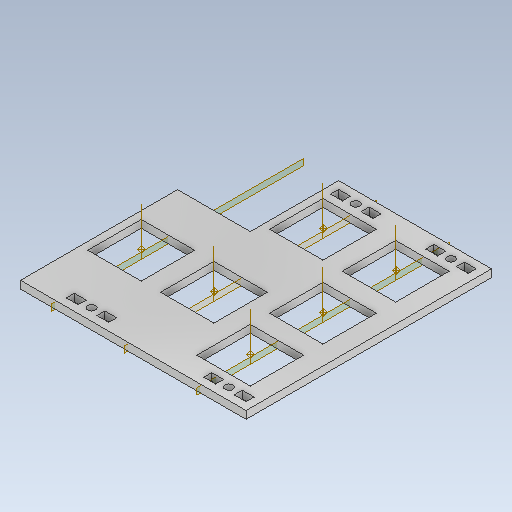
# Autodesk Inventor part: tc_base_plate
Saved by Autodesk Inventor 2020.1 (Build 241239000, 239)
## iProperties
Created: 2019-07-03
Part Number: tc_base_plate
Material: Acier inoxydable
Document SubType Name: Modeling
Designer: Thibault
Density: 8 g/cm^3
Appearance: Aluminium - Poli
Mass: 33.3223 g
Surface Area: 56.2435 cm^2
Volume: 4.16528 cm^3
tc_base_width: 59,100 mm
tc_base_back_width: 40,050 mm
tc_base_support_dist: 56,100 mm
Author: Thibault
Autodesk Inventor part; units mm, degrees
ref_plane "YZ Plane" through (0, 0, 0) normal (1, 0, 0) x (0, 1, 0)
ref_plane "XZ Plane" through (0, 0, 0) normal (0, 1, 0) x (-1, 0, 0)
ref_plane "XY Plane" through (0, 0, 0) normal (0, 0, 1) x (1, 0, 0)
sketch "screw_anchor" plane through (0, 0, 0) normal (0, 0, 1) x (1, 0, 0)
  point P0 (61.1245, 15.5217)
  dimension "d155" = 14
  dimension "d156" = 19.05
  dimension "d157" = 19.05
  dimension "d158" = 19.05
  dimension "d159" = 28.575
  dimension "d160" = 19.05
  dimension "d161" = 2
  dimension "d162" = 2
  dimension "d163" = 2
  dimension "d164" = 2
  dimension "d165" = 2
  dimension "d166" = 1
  dimension "d167" = 5
  dimension "d168" = 5
  dimension "d169" = 4
  dimension "tc_base_support_dist" = 56.1
sketch "anchor" plane through (0, 0, 0) normal (0, 0, 1) x (1, 0, 0)
  circle A0 centre (94.2814, 48.5827) radius 0.85
  line L0 (91.2814, 49.5827) -> (87.2814, 49.5827)
  line L1 (87.2814, 49.5827) -> (87.2814, 47.5827)
  line L2 (87.2814, 47.5827) -> (91.2814, 47.5827)
  line L3 (91.2814, 47.5827) -> (91.2814, 49.5827)
  line L4 (101.2814, 49.5827) -> (97.2814, 49.5827)
  line L5 (97.2814, 49.5827) -> (97.2814, 47.5827)
  line L6 (97.2814, 47.5827) -> (101.2814, 47.5827)
  line L7 (101.2814, 47.5827) -> (101.2814, 49.5827)
  line L8 (91.2814, 49.5827) -> (97.2814, 47.5827) construction
  line L9 (97.2814, 49.5827) -> (91.2814, 47.5827) construction
  line L10 (87.2814, 51.1827) -> (101.2814, 51.1827)
  point P0 (103.5798, 50.1132)
  point P1 (94.2814, 48.5827)
  dimension "tc_base_support_dist" = 56.1
  dimension "d226" = 1.7
  dimension "d230" = 4
  dimension "d231" = 2
  dimension "d237" = 4
  dimension "d245" = 1.6
  dimension "d247" = 6
  measures "d226" diameter of A0
  measures "d230" distance of L2.end L1.end
  measures "d231" distance of L1.end L0.end
  measures "d237" distance of L6.end L5.end
  measures "d245" distance between parallel lines of L0 L10
  measures "d247" distance between parallel lines of L5 L3
sketch "Anchor (screw side)" plane through (0, 0, 0) normal (0, 0, 1) x (1, 0, 0)
  circle A0 centre (93.7216, 50.3096) radius 1.05
  line L0 (91.2716, 51.3596) -> (88.1716, 51.3596)
  line L1 (88.1716, 51.3596) -> (88.1716, 49.2596)
  line L2 (88.1716, 49.2596) -> (91.2716, 49.2596)
  line L3 (91.2716, 49.2596) -> (91.2716, 51.3596)
  line L4 (99.2716, 51.3596) -> (96.1716, 51.3596)
  line L5 (96.1716, 51.3596) -> (96.1716, 49.2596)
  line L6 (96.1716, 49.2596) -> (99.2716, 49.2596)
  line L7 (99.2716, 49.2596) -> (99.2716, 51.3596)
  line L8 (91.2716, 51.3596) -> (96.1716, 49.2596) construction
  line L9 (96.1716, 51.3596) -> (91.2716, 49.2596) construction
  line L10 (86.1716, 53.3596) -> (101.2716, 53.3596) construction
  line L11 (101.2716, 53.3596) -> (101.2716, 47.2596) construction
  line L12 (101.2716, 47.2596) -> (86.1716, 47.2596) construction
  line L13 (86.1716, 47.2596) -> (86.1716, 53.3596) construction
  point P0 (103.5798, 50.1132)
  dimension "d27" = 2.1
  dimension "d28" = 3.1
  dimension "d29" = 2.1
  dimension "d32" = 4.9
  dimension "d34" = 2
  dimension "d35" = 2
  dimension "d36" = 2
  dimension "d37" = 2
  measures "d27" diameter of A0
  measures "d28" distance of L2.end L1.end
  measures "d29" distance of L1.end L0.end
  measures "d32" distance between parallel lines of L5 L3
  measures "d34" distance between parallel lines of L0 L10
  measures "d35" distance between parallel lines of L12 L2
  measures "d36" distance between parallel lines of L11 L7
  measures "d37" distance between parallel lines of L13 L1
sketch "Anchor (nut side)" plane through (0, 0, 0) normal (0, 0, 1) x (1, 0, 0)
  line L0 (10, 0) -> (8.55, 0)
  line L1 (8.55, 0) -> (8.55, -2)
  line L2 (8.55, -2) -> (9.35, -2)
  line L3 (9.35, -2) -> (9.35, -4)
  line L4 (5.65, -4) -> (5.65, -2)
  line L5 (5.65, -2) -> (6.45, -2)
  line L6 (6.45, -2) -> (6.45, 0)
  line L7 (6.45, 0) -> (5, 0)
  line L8 (2, 0) -> (2, 2)
  line L9 (2, 0) -> (3, 0) construction
  line L10 (2, 2) -> (5, 2)
  line L11 (5, 2) -> (5, 0)
  line L12 (10, 0) -> (10, 2)
  line L13 (10, 2) -> (13, 2)
  line L14 (13, 2) -> (13, 0)
  line L15 (0, 0) -> (2, 0)
  line L16 (13, 0) -> (15, 0)
  line L17 (5.65, -4) -> (6.45, -4)
  line L18 (9.35, -4) -> (8.55, -4)
  line L19 (6.45, -4) -> (6.45, -6.25)
  line L20 (8.55, -4) -> (8.55, -6.25)
  line L21 (6.7, -6.5) -> (7.5, -6.5)
  arc A0 (6.45, -6.25) -> (6.7, -6.5) centre (6.7, -6.25) ccw
  arc A1 (8.3, -6.5) -> (8.55, -6.25) centre (8.3, -6.25) ccw
  line L22 (7.5, -6.5) -> (8.3, -6.5)
  line L23 (7.5, -3.8983) -> (7.5, -9.959) construction
  point P0 (9.1321, -0.6227)
  point P1 (6.45, -6.5)
  point P2 (8.55, -6.5)
  dimension "d3" = 2
  dimension "d7" = 5
  dimension "d10" = 1.45
  dimension "d11" = 2
  dimension "d12" = 0.8
  dimension "d13" = 2
  dimension "d14" = 0.8
  dimension "d15" = 2.1
  dimension "d18" = 2
  dimension "d19" = 0.8
  dimension "d20" = 0.8
  dimension "d21" = 2.5
  dimension "d22" = 2.5
  dimension "d23" = 2.1
  dimension "d38" = 2
  dimension "d39" = 0.25
  dimension "d120" = 3
  measures "d3" distance of L15.start L8.start
  measures "d7" distance of L7.end L0.start
  measures "d10" distance of L0.start L0.end
  measures "d11" distance of L0.end L1.end
  measures "d12" distance of L1.end L2.end
  measures "d13" distance of L2.end L3.end
  measures "d14" distance of L4.end L5.end
  measures "d15" distance of L6.end L0.end
  measures "d18" distance of L14.end L16.end
  measures "d19" distance of L4.start L17.end
  measures "d20" distance of L3.end L18.end
  measures "d21" distance of L17.end point (6.45, -6.5)
  measures "d22" distance of L18.end point (8.55, -6.5)
  measures "d23" distance of L17.end L18.end
  measures "d38" distance between parallel lines of L15 L10
  measures "d39" radius of A0
  measures "d120" distance of L8.end L10.end
sketch "Screwless anchor (male)" plane through (0, 0, 0) normal (0, 0, 1) x (1, 0, 0)
  line L0 (2, 0) -> (2, 2)
  line L1 (2, 0) -> (3, 0) construction
  line L2 (2, 2) -> (5, 2)
  line L3 (5, 2) -> (5, 0)
  line L4 (10, 0) -> (10, 2)
  line L5 (10, 2) -> (13, 2)
  line L6 (13, 2) -> (13, 0)
  line L7 (0, 0) -> (2, 0)
  line L8 (13, 0) -> (15, 0)
  line L9 (5, 0) -> (10, 0)
  point P0 (9.1321, -0.6227)
  dimension "d81" = 2
  dimension "d83" = 5
  dimension "d92" = 2
  dimension "d100" = 2
  dimension "d119" = 3
  measures "d81" distance of L7.start L0.start
  measures "d83" distance of L3.end L4.start
  measures "d92" distance of L6.end L8.end
  measures "d100" distance between parallel lines of L7 L2
  measures "d119" distance of L0.end L2.end
sketch "Screwless anchor (female)" plane through (0, 0, 0) normal (0, 0, 1) x (1, 0, 0)
  line L0 (91.7814, 51.7592) -> (88.6814, 51.7592)
  line L1 (88.6814, 51.7592) -> (88.6814, 49.6592)
  line L2 (88.6814, 49.6592) -> (91.7814, 49.6592)
  line L3 (91.7814, 49.6592) -> (91.7814, 51.7592)
  line L4 (99.7814, 51.7592) -> (96.6814, 51.7592)
  line L5 (96.6814, 51.7592) -> (96.6814, 49.6592)
  line L6 (96.6814, 49.6592) -> (99.7814, 49.6592)
  line L7 (99.7814, 49.6592) -> (99.7814, 51.7592)
  line L8 (86.6814, 53.7592) -> (101.7814, 53.7592) construction
  line L9 (101.7814, 53.7592) -> (101.7814, 47.6592) construction
  line L10 (101.7814, 47.6592) -> (86.6814, 47.6592) construction
  line L11 (86.6814, 47.6592) -> (86.6814, 53.7592) construction
  point P0 (103.5798, 50.1132)
  dimension "d106" = 3.1
  dimension "d107" = 2.1
  dimension "d108_1" = 3.1
  dimension "d109_1" = 4.9
  dimension "d110_1" = 2
  dimension "d111_1" = 2
  dimension "d112" = 2
  dimension "d113" = 2
  measures "d106" distance of L2.end L1.end
  measures "d107" distance of L1.end L0.end
  measures "d108_1" distance of L6.end L5.end
  measures "d109_1" distance between parallel lines of L5 L3
  measures "d110_1" distance between parallel lines of L0 L8
  measures "d111_1" distance between parallel lines of L10 L2
  measures "d112" distance between parallel lines of L9 L7
  measures "d113" distance between parallel lines of L11 L1
sketch "Esquisse2" plane through (0, 0, 0) normal (0, 1, 0) x (-1, 0, 0)
  line L0 (17.4004, -3.6293) -> (3.4004, -3.6293)
  line L1 (3.4004, -3.6293) -> (3.4004, 10.3707)
  line L2 (3.4004, 10.3707) -> (17.4004, 10.3707)
  line L3 (17.4004, 10.3707) -> (17.4004, -3.6293)
  line L4 (17.4004, -41.7293) -> (3.4004, -41.7293)
  line L5 (3.4004, -41.7293) -> (3.4004, -27.7293)
  line L6 (3.4004, -27.7293) -> (17.4004, -27.7293)
  line L7 (17.4004, -27.7293) -> (17.4004, -41.7293)
  line L8 (17.4004, -22.6793) -> (3.4004, -22.6793)
  line L9 (3.4004, -22.6793) -> (3.4004, -8.6793)
  line L10 (3.4004, -8.6793) -> (17.4004, -8.6793)
  line L11 (17.4004, -8.6793) -> (17.4004, -22.6793)
  line L12 (36.4504, -41.7293) -> (22.4504, -41.7293)
  line L13 (22.4504, -41.7293) -> (22.4504, -27.7293)
  line L14 (22.4504, -27.7293) -> (36.4504, -27.7293)
  line L15 (36.4504, -27.7293) -> (36.4504, -41.7293)
  line L16 (36.4504, -13.1543) -> (22.4504, -13.1543)
  line L17 (22.4504, -13.1543) -> (22.4504, 0.8457)
  line L18 (22.4504, 0.8457) -> (36.4504, 0.8457)
  line L19 (36.4504, 0.8457) -> (36.4504, -13.1543)
  line L20 (55.5004, -13.1543) -> (41.5004, -13.1543)
  line L21 (41.5004, -13.1543) -> (41.5004, 0.8457)
  line L22 (41.5004, 0.8457) -> (55.5004, 0.8457)
  line L23 (55.5004, 0.8457) -> (55.5004, -13.1543)
  line L24 (57.5004, -24.6793) -> (38.4504, -24.6793)
  line L25 (38.4504, -24.6793) -> (38.4504, -47.8293)
  line L26 (38.4504, -47.8293) -> (-1.5996, -47.8293)
  line L27 (-1.5996, -47.8293) -> (-1.5996, 16.4707)
  line L28 (57.5004, -24.6793) -> (57.5004, 16.4707)
  line L29 (57.5004, 16.4707) -> (-1.5996, 16.4707)
  circle A0 centre (41.9504, 13.4207) radius 1.05
  line L30 (39.5004, 14.4707) -> (36.4004, 14.4707)
  line L31 (36.4004, 14.4707) -> (36.4004, 12.3707)
  line L32 (36.4004, 12.3707) -> (39.5004, 12.3707)
  line L33 (39.5004, 12.3707) -> (39.5004, 14.4707)
  line L34 (47.5004, 14.4707) -> (44.4004, 14.4707)
  line L35 (44.4004, 14.4707) -> (44.4004, 12.3707)
  line L36 (44.4004, 12.3707) -> (47.5004, 12.3707)
  line L37 (47.5004, 12.3707) -> (47.5004, 14.4707)
  line L38 (39.5004, 14.4707) -> (44.4004, 12.3707) construction
  line L39 (44.4004, 14.4707) -> (39.5004, 12.3707) construction
  line L40 (34.4004, 16.4707) -> (49.5004, 16.4707) construction
  line L41 (49.5004, 16.4707) -> (49.5004, 10.3707) construction
  line L42 (49.5004, 10.3707) -> (34.4004, 10.3707) construction
  line L43 (34.4004, 10.3707) -> (34.4004, 16.4707) construction
  circle A1 centre (5.9504, 13.4207) radius 1.05
  line L44 (3.5004, 14.4707) -> (0.4004, 14.4707)
  line L45 (0.4004, 14.4707) -> (0.4004, 12.3707)
  line L46 (0.4004, 12.3707) -> (3.5004, 12.3707)
  line L47 (3.5004, 12.3707) -> (3.5004, 14.4707)
  line L48 (11.5004, 14.4707) -> (8.4004, 14.4707)
  line L49 (8.4004, 14.4707) -> (8.4004, 12.3707)
  line L50 (8.4004, 12.3707) -> (11.5004, 12.3707)
  line L51 (11.5004, 12.3707) -> (11.5004, 14.4707)
  line L52 (3.5004, 14.4707) -> (8.4004, 12.3707) construction
  line L53 (8.4004, 14.4707) -> (3.5004, 12.3707) construction
  line L54 (-1.5996, 16.4707) -> (13.5004, 16.4707) construction
  line L55 (13.5004, 16.4707) -> (13.5004, 10.3707) construction
  line L56 (13.5004, 10.3707) -> (-1.5996, 10.3707) construction
  line L57 (-1.5996, 10.3707) -> (-1.5996, 16.4707) construction
  circle A2 centre (5.9504, -44.7793) radius 1.05
  line L58 (3.5004, -43.7293) -> (0.4004, -43.7293)
  line L59 (0.4004, -43.7293) -> (0.4004, -45.8293)
  line L60 (0.4004, -45.8293) -> (3.5004, -45.8293)
  line L61 (3.5004, -45.8293) -> (3.5004, -43.7293)
  line L62 (11.5004, -43.7293) -> (8.4004, -43.7293)
  line L63 (8.4004, -43.7293) -> (8.4004, -45.8293)
  line L64 (8.4004, -45.8293) -> (11.5004, -45.8293)
  line L65 (11.5004, -45.8293) -> (11.5004, -43.7293)
  line L66 (3.5004, -43.7293) -> (8.4004, -45.8293) construction
  line L67 (8.4004, -43.7293) -> (3.5004, -45.8293) construction
  line L68 (-1.5996, -41.7293) -> (13.5004, -41.7293) construction
  line L69 (13.5004, -41.7293) -> (13.5004, -47.8293) construction
  line L70 (13.5004, -47.8293) -> (-1.5996, -47.8293) construction
  line L71 (-1.5996, -47.8293) -> (-1.5996, -41.7293) construction
  circle A3 centre (30.9004, -44.7793) radius 1.05
  line L72 (28.4504, -43.7293) -> (25.3504, -43.7293)
  line L73 (25.3504, -43.7293) -> (25.3504, -45.8293)
  line L74 (25.3504, -45.8293) -> (28.4504, -45.8293)
  line L75 (28.4504, -45.8293) -> (28.4504, -43.7293)
  line L76 (36.4504, -43.7293) -> (33.3504, -43.7293)
  line L77 (33.3504, -43.7293) -> (33.3504, -45.8293)
  line L78 (33.3504, -45.8293) -> (36.4504, -45.8293)
  line L79 (36.4504, -45.8293) -> (36.4504, -43.7293)
  line L80 (28.4504, -43.7293) -> (33.3504, -45.8293) construction
  line L81 (33.3504, -43.7293) -> (28.4504, -45.8293) construction
  line L82 (23.3504, -41.7293) -> (38.4504, -41.7293) construction
  line L83 (38.4504, -41.7293) -> (38.4504, -47.8293) construction
  line L84 (38.4504, -47.8293) -> (23.3504, -47.8293) construction
  line L85 (23.3504, -47.8293) -> (23.3504, -41.7293) construction
  point P0 (39.3203, -53.3777)
  point P1 (31.897, -47.8293)
  point P2 (1.2703, -53.3777)
  dimension "tc_base_support_dist" = 56.1
  dimension "d108" = 14
  dimension "d109" = 19.05
  dimension "d110" = 19.05
  dimension "d111" = 19.05
  dimension "d114" = 19.05
  dimension "d123" = 2
  dimension "d181" = 5
  dimension "d190" = 2
  dimension "d258" = 10
  dimension "d260" = 2
  dimension "d263" = 2
  dimension "d269" = 28.575
  dimension "d275" = 2
  constraints: 60 end point, 12 horizontal, 12 parallel, 11 equal length, 7 perpendicular, 6 vertical, 5 collinear, 3 point on line
  measures "d108" distance of L1.end L2.end
  measures "d109" distance of L8.end L4.end
  measures "d110" distance of L0.end L8.end
  measures "d111" distance of L4.start L12.start
  measures "d114" distance of L18.end L22.end
  measures "d123" distance between parallel lines of L8 L24
  measures "d181" distance between parallel lines of L27 L5
  measures "d190" distance between parallel lines of L28 L23
  measures "d269" distance between parallel lines of L16 L12
  measures "d275" distance between parallel lines of L25 L15
extrude "Base" add sketch "Esquisse2" along normal blind 2
ref_plane "Plan de construction4" through (-10.4004, 0, -41.7293) normal (-1, 0, 0) x (0, 0, 1)
ref_plane "Plan de construction5" through (-29.4504, 0, -27.7293) normal (1, 0, 0) x (0, 0, -1)
ref_plane "Plan de construction6" through (-48.5004, 0, -13.1543) normal (-1, 0, 0) x (0, 0, 1)
derived "shared_parameters.ipt"
